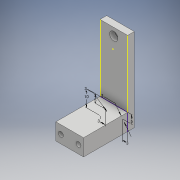
# Autodesk Inventor part: armpart1
Saved by Autodesk Inventor 2018.3 (Build 223284000, 284)
## iProperties
Created: 2019-11-01
Part Number: armpart1
Material: 一般
Document SubType Name: Modeling
Designer: Eiji Nishizawa
Density: 1 g/cm^3
Appearance: 既定
Author: Eiji Nishizawa
Autodesk Inventor part; units mm, degrees
ref_plane "YZ Plane" through (0, 0, 0) normal (1, 0, 0) x (0, 1, 0)
ref_plane "XZ Plane" through (0, 0, 0) normal (0, 1, 0) x (-1, 0, 0)
ref_plane "XY Plane" through (0, 0, 0) normal (0, 0, 1) x (1, 0, 0)
sketch "スケッチ1" plane through (0, 0, 0) normal (0, 1, 0) x (-1, 0, 0)
  line L0 (7.8325, 11.4458) -> (-8.7675, 11.4458)
  line L1 (-8.7675, 11.4458) -> (-8.7675, -38.5542)
  line L2 (-8.7675, -38.5542) -> (7.8325, -38.5542)
  line L3 (7.8325, -38.5542) -> (7.8325, 11.4458)
  circle A0 centre (-0.4675, 6.9458) radius 2.5
  point P0 (0, 0)
  dimension "d0" = 16.6
  dimension "d1" = 5
  dimension "d2" = 8.3
  dimension "d3" = 8.3
  dimension "d4" = 4.5
  dimension "d5" = 2
  dimension "d6" = 50
  constraints: 8 end point, 2 parallel, 1 centre point, 1 horizontal, 1 perpendicular
  measures "d0" distance of L0.start L0.end
  measures "d1" diameter of A0
  measures "d2" distance from line of L3 A0.centre
  measures "d3" distance from line of L1 A0.centre
  measures "d4" distance from line of L0 A0.centre
  measures "d5" distance edge to line of A0 L0
  measures "d6" distance of L2.end L0.start
extrude "押し出し1" add sketch "スケッチ1" along normal blind 3
sketch "スケッチ2" plane through (0, 3, 0) normal (0, 1, 0) x (1, 0, 0)
  line L0 (-7.8325, 38.5542) -> (-7.8325, -11.4458) projected
  line L1 (8.7675, -11.4458) -> (8.7675, 38.5542) projected
  line L2 (-7.8325, -11.4458) -> (8.7675, -11.4458)
  line L3 (8.7675, -11.4458) -> (8.7675, 38.5542)
  line L4 (8.7675, 38.5542) -> (-7.8325, 38.5542)
  line L5 (-7.8325, 38.5542) -> (-7.8325, -11.4458)
  circle A0 centre (0.4675, -6.9458) radius 1.5
  circle A1 centre (0.4675, -6.9458) radius 2.5 projected
  point P0 (0, 0)
  dimension "d9" = 3
  constraints: 8 end point, 2 parallel, 1 centre point, 1 concentric, 1 horizontal, 1 perpendicular
  measures "d9" diameter of A0
extrude "押し出し2" add sketch "スケッチ2" along normal blind 1 contours L4 L1 L2 L0 | A1
sketch "スケッチ3" plane through (0, 0, 0) normal (0, -1, 0) x (1, 0, 0)
  line L0 (-7.8325, -38.5542) -> (-7.8325, 11.4458) projected
  line L1 (8.7675, 11.4458) -> (8.7675, -38.5542) projected
  line L2 (-7.8325, -38.5542) -> (8.7675, -38.5542)
  line L3 (8.7675, -38.5542) -> (8.7675, -28.5542)
  line L4 (8.7675, -28.5542) -> (-7.8325, -28.5542)
  line L5 (-7.8325, -28.5542) -> (-7.8325, -38.5542)
  circle A0 centre (5.7675, -33.5542) radius 1.5
  circle A1 centre (-4.8325, -33.5542) radius 1.5
  point P0 (0, 0)
  dimension "d12" = 10
  dimension "d13" = 5
  dimension "d14" = 5
  dimension "d15" = 3
  dimension "d16" = 3
  dimension "d17" = 3
  dimension "d18" = 3
  constraints: 8 end point, 2 centre point, 2 parallel, 1 horizontal, 1 perpendicular, 1 point on line
  measures "d12" distance between parallel lines of L2 L4
  measures "d13" distance from line of L4 A1.centre
  measures "d14" distance from line of L4 A0.centre
  measures "d15" diameter of A0
  measures "d16" diameter of A1
  measures "d17" distance from line of L0 A1.centre
  measures "d18" distance from line of L1 A0.centre
extrude "押し出し3" add sketch "スケッチ3" along normal blind 26.5
extrude "押し出し4" cut sketch "スケッチ3" against normal blind 21 contours A0 | A1
